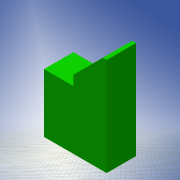
# Autodesk Inventor part: _WT_Aufnahme1
Saved by Autodesk Inventor 2025.1 (Build 291241000, 241)
## iProperties
Created: 2025-05-02
Part Number: _WT_Aufnahme1
Material: Generisch
Document SubType Name: Modeling
Designer: RP
Density: 1 g/cm^3
Appearance: Vorgabe
Author: RP
Autodesk Inventor part; units mm, degrees
ref_plane "YZ Plane" through (0, 0, 0) normal (1, 0, 0) x (0, 1, 0)
ref_plane "XZ Plane" through (0, 0, 0) normal (0, 1, 0) x (-1, 0, 0)
ref_plane "XY Plane" through (0, 0, 0) normal (0, 0, 1) x (1, 0, 0)
sketch "Skizze1" plane through (0, 0, 0) normal (0, 0, 1) x (1, 0, 0)
  line L0 (76.2299, 50.7181) -> (91.2299, 50.7181)
  line L1 (91.2299, 50.7181) -> (91.2299, 55.7181)
  line L2 (91.2299, 55.7181) -> (106.2299, 70.7181)
  line L3 (106.2299, 70.7181) -> (108.2299, 70.7181)
  line L4 (108.2299, 70.7181) -> (108.2299, 20.7181)
  line L5 (108.2299, 20.7181) -> (76.2299, 20.7181)
  line L6 (76.2299, 20.7181) -> (76.2299, 50.7181)
  point P0 (0, 0)
  dimension "d0" = 30
  dimension "d1" = 15
  dimension "d2" = 45
  dimension "d5" = 50
  dimension "d6" = 5
  dimension "d7" = 32
  constraints: 14 end point, 4 perpendicular, 1 horizontal, 1 parallel
  measures "d0" distance of L5.end L0.start
  measures "d1" distance of L0.start L0.end
  measures "d2" angle of L1 L2
  measures "d5" distance of L3.end L4.end
  measures "d6" distance of L0.end L1.end
  measures "d7" distance of L4.end L5.end
extrude "Extrusion1" add sketch "Skizze1" along normal mid plane 15
